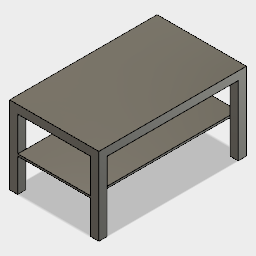
Lack (Autodesk Fusion 360 design; units mm, degrees)
Autodesk Fusion 360 part; units mm, degrees
sketch "Sketch1" plane through (0, 0, 0) normal (0, 1, 0) x (1, 0, 0)
  line L0 (0, 0) -> (50.8, 0)
  line L1 (50.8, 0) -> (50.8, -50.8)
  line L2 (50.8, -50.8) -> (0, -50.8)
  line L3 (0, -50.8) -> (0, 0)
  line L4 (0, -850.9) -> (50.8, -850.9)
  line L5 (50.8, -850.9) -> (50.8, -901.7)
  line L6 (50.8, -901.7) -> (0, -901.7)
  line L7 (0, -901.7) -> (0, -850.9)
  line L8 (0, -50.8) -> (0, 0)
  line L9 (50.8, 0) -> (50.8, -50.8)
  line L10 (0, 0) -> (50.8, 0)
  line L11 (50.8, -50.8) -> (0, -50.8)
  line L12 (546.1, -50.3836) -> (495.3, -50.3836)
  line L13 (546.1, 0.4164) -> (546.1, -50.3836)
  line L14 (495.3, 0.4164) -> (546.1, 0.4164)
  line L15 (495.3, -50.3836) -> (495.3, 0.4164)
  line L16 (495.3, -850.9) -> (546.1, -850.9)
  line L17 (546.1, -850.9) -> (546.1, -901.7)
  line L18 (546.1, -901.7) -> (495.3, -901.7)
  line L19 (495.3, -901.7) -> (495.3, -850.9)
  dimension "d1" = 50.8
  dimension "d2" = 50.8
  dimension "d3" = 50.8
  dimension "d4" = 50.8
  dimension "d5" = 800.1
  dimension "d6" = 50.8
  dimension "d7" = 50.8
  dimension "d8" = 50.8
  dimension "d9" = 50.8
  dimension "d10" = 444.5
  dimension "d11" = 50.8
  dimension "d12" = 50.8
  measures "d1" distance of L0.end L1.end
  measures "d2" distance of L0.start L0.end
  measures "d3" distance of L4.end L5.end
  measures "d4" distance of L5.end L6.end
  measures "d5" distance of L2 L4
  measures "d6" distance of L0.end L1.end
  measures "d7" distance of L0.end L0.start
  measures "d8" distance of L12.start L13.start
  measures "d9" distance of L14.start L13.start
  measures "d10" distance of L9 L15
  measures "d11" distance of L17.end L18.end
  measures "d12" distance of L16.start L18.end
extrude "Extrude1" add sketch "Sketch1" along normal blind 425.45 makes body 1 at (512.2333, 141.8167, 850.9) makes body 2 at (529.1667, 141.8167, 50.3836) makes body 3 at (16.9333, 141.8167, 850.9) makes body 4 at (16.9333, 141.8167, 0)
sketch "Sketch2" plane through (0, 425.45, 0) normal (0, 1, 0) x (-1, 0, 0)
  line L0 (0, 901.7) -> (-50.8, 901.7)
  line L1 (-50.8, 901.7) -> (-50.8, 850.9)
  line L2 (-50.8, 850.9) -> (0, 850.9)
  line L3 (0, 850.9) -> (0, 901.7)
  line L4 (0, 901.7) -> (-546.1, 901.7)
  line L5 (-546.1, 901.7) -> (-546.1, -0.4164)
  line L6 (-546.1, -0.4164) -> (0, -0.4164)
  line L7 (0, -0.4164) -> (0, 901.7)
  point P0 (-546.1, -0.4164)
extrude "Extrude2" add sketch "Sketch2" along normal blind 50.8 bodies 1 2 3 4
sketch "Sketch3" plane through (0, 0, 901.7) normal (0, 0, 1) x (1, 0, 0)
  line L0 (495.3, 0) -> (546.1, 0)
  line L1 (546.1, 0) -> (546.1, 476.25)
  line L2 (546.1, 476.25) -> (0, 476.25)
  line L3 (0, 476.25) -> (0, 0)
  line L4 (0, 0) -> (50.8, 0)
  line L5 (50.8, 0) -> (50.8, 425.45)
  line L6 (50.8, 425.45) -> (495.3, 425.45)
  line L7 (495.3, 425.45) -> (495.3, 0)
  line L8 (50.8, 215.9) -> (495.3, 215.9)
  line L9 (495.3, 215.9) -> (495.3, 203.2)
  line L10 (495.3, 203.2) -> (50.8, 203.2)
  line L11 (50.8, 203.2) -> (50.8, 215.9)
  dimension "d22" = 444.5
  dimension "d23" = 12.7
  dimension "d24" = 203.2
  measures "d22" distance of L8.start L8.end
  measures "d23" distance of L8.start L10.end
  measures "d24" distance of L4 L10
extrude "Extrude3" add sketch "Sketch3" against normal blind 901.7 contours L5 L7 L8 L9 L10 L11 bodies 1
